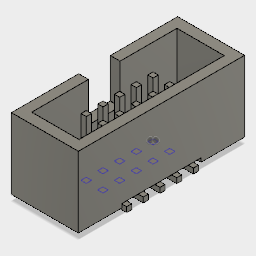
Gadgeteer Socket v1 (Autodesk Fusion 360 design; units mm, degrees)
Autodesk Fusion 360 part; units mm, degrees
sketch "Sketch1" plane through (0, 0, 0) normal (0, 1, 0) x (1, 0, 0)
  line L0 (2.55, 6.325) -> (-2.55, 6.325)
  line L1 (-2.55, 6.325) -> (-2.55, -6.325)
  line L2 (-2.55, -6.325) -> (2.55, -6.325)
  line L3 (2.55, -6.325) -> (2.55, 6.325)
  line L4 (2.55, 6.325) -> (-2.55, -6.325) construction
  line L5 (-2.55, 6.325) -> (2.55, -6.325) construction
  line L6 (1.8, 5.525) -> (-1.8, 5.525)
  line L7 (-1.8, 5.525) -> (-1.8, -5.525)
  line L8 (-1.8, -5.525) -> (1.8, -5.525)
  line L9 (1.8, -5.525) -> (1.8, 5.525)
  line L10 (1.8, 5.525) -> (-1.8, -5.525) construction
  line L11 (-1.8, 5.525) -> (1.8, -5.525) construction
  dimension "d1" = 12.65
  dimension "d2" = 5.1
  dimension "d3" = 3.6
  dimension "d4" = 11.05
  constraint perpendicular L0 L1
  constraint parallel L0 L2
  constraint parallel L1 L3
  constraint horizontal L0
  constraint coincident L4
  constraint coincident L5
  constraint perpendicular L6 L7
  constraint parallel L6 L8
  constraint parallel L7 L9
  constraint horizontal L6
  constraint coincident L10
  constraint coincident L11
extrude "Extrude1" add sketch "Sketch1" along normal blind 5.4 makes body 1
sketch "Sketch2" plane through (0, 5.4, 0) normal (0, 1, 0) x (-1, 0, 0)
  line L0 (-1.8, -5.525) -> (-1.8, 5.525)
  line L1 (-1.8, 5.525) -> (1.8, 5.525)
  line L2 (1.8, 5.525) -> (1.8, -5.525)
  line L3 (1.8, -5.525) -> (-1.8, -5.525)
  line L4 (-2.55, 6.325) -> (-2.55, -6.325)
  line L5 (-2.55, -6.325) -> (2.55, -6.325)
  line L6 (2.55, -6.325) -> (2.55, 6.325)
  line L7 (2.55, 6.325) -> (-2.55, 6.325)
  line L8 (1.8, 0) -> (2.55, 0)
  line L9 (1.8, -1.2) -> (2.55, -1.2)
  line L10 (2.55, -1.2) -> (2.55, 1.2)
  line L11 (2.55, 1.2) -> (1.8, 1.2)
  line L12 (1.8, 1.2) -> (1.8, -1.2)
  line L13 (1.8, -1.2) -> (2.55, 1.2) construction
  line L14 (2.55, -1.2) -> (1.8, 1.2) construction
  dimension "d7" = 2.4
  constraint midpoint L2
  constraint midpoint L6
  constraint perpendicular L9 L10
  constraint parallel L9 L11
  constraint parallel L10 L12
  constraint horizontal L9
  constraint coincident L13
  constraint coincident L14
  constraint midpoint L8
extrude "Extrude2" cut sketch "Sketch2" against normal blind 3 contours L2 L6 L8 L9 L10 L12 | L2 L6 L8 L10 L11 L12 bodies 1
extrude "Extrude3" add sketch "Sketch1" along normal blind 1 contours L6 L7 L8 L9 bodies 1
sketch "Sketch3" plane through (0, 0, 0) normal (0, 1, 0) x (1, 0, 0)
  line L0 (-0.835, 2.74) -> (-0.435, 2.74)
  line L1 (-0.435, 2.74) -> (-0.435, 2.34)
  line L2 (-0.435, 2.34) -> (-0.835, 2.34)
  line L3 (-0.835, 2.34) -> (-0.835, 2.74)
  line L4 (0.835, 2.74) -> (0.835, 2.34)
  line L5 (0.435, 2.74) -> (0.835, 2.74)
  line L6 (0.835, 2.34) -> (0.435, 2.34)
  line L7 (0.435, 2.34) -> (0.435, 2.74)
  line L8 (-0.435, 1.47) -> (-0.435, 1.07)
  line L9 (-0.835, 1.47) -> (-0.435, 1.47)
  line L10 (-0.435, 1.07) -> (-0.835, 1.07)
  line L11 (-0.835, 1.07) -> (-0.835, 1.47)
  line L12 (0.835, 1.47) -> (0.835, 1.07)
  line L13 (0.435, 1.47) -> (0.835, 1.47)
  line L14 (0.835, 1.07) -> (0.435, 1.07)
  line L15 (0.435, 1.07) -> (0.435, 1.47)
  line L16 (-0.435, 0.2) -> (-0.435, -0.2)
  line L17 (-0.835, 0.2) -> (-0.435, 0.2)
  line L18 (-0.435, -0.2) -> (-0.835, -0.2)
  line L19 (-0.835, -0.2) -> (-0.835, 0.2)
  line L20 (0.835, 0.2) -> (0.835, -0.2)
  line L21 (0.435, 0.2) -> (0.835, 0.2)
  line L22 (0.835, -0.2) -> (0.435, -0.2)
  line L23 (0.435, -0.2) -> (0.435, 0.2)
  line L24 (-0.435, -1.07) -> (-0.435, -1.47)
  line L25 (-0.835, -1.07) -> (-0.435, -1.07)
  line L26 (-0.435, -1.47) -> (-0.835, -1.47)
  line L27 (-0.835, -1.47) -> (-0.835, -1.07)
  line L28 (0.835, -1.07) -> (0.835, -1.47)
  line L29 (0.435, -1.07) -> (0.835, -1.07)
  line L30 (0.835, -1.47) -> (0.435, -1.47)
  line L31 (0.435, -1.47) -> (0.435, -1.07)
  line L32 (-0.435, -2.34) -> (-0.435, -2.74)
  line L33 (-0.835, -2.34) -> (-0.435, -2.34)
  line L34 (-0.435, -2.74) -> (-0.835, -2.74)
  line L35 (-0.835, -2.74) -> (-0.835, -2.34)
  line L36 (0.835, -2.34) -> (0.835, -2.74)
  line L37 (0.435, -2.34) -> (0.835, -2.34)
  line L38 (0.835, -2.74) -> (0.435, -2.74)
  line L39 (0.435, -2.74) -> (0.435, -2.34)
  dimension "d12" = 0.4
  dimension "d13" = 0.4
  dimension "d16" = 1.27
  dimension "d17" = -5.08
  dimension "d20" = 2.54
  dimension "d21" = 0.635
  constraint horizontal L0
  constraint vertical L1
  constraint horizontal L2
  constraint vertical L3
  constraint midpoint L3
  constraint midpoint L0
extrude "Extrude4" add sketch "Sketch3" along normal blind 4.4 separate body makes body 2 at (0.5683, 1.4667, -0.2) makes body 3 at (0.835, 1.4667, -1.3367) makes body 4 at (0.835, 1.4667, 1.2033) makes body 5 at (-0.435, 1.4667, 2.4733) makes body 6 at (-0.7017, 1.4667, -0.2) makes body 7 at (0.835, 1.4667, 2.4733) makes body 8 at (-0.435, 1.4667, 1.2033) makes body 9 at (-0.435, 1.4667, -1.3367) makes body 10 at (-0.7017, 1.4667, -2.74) makes body 11 at (0.5683, 1.4667, -2.74)
extrude "Extrude5" add sketch "Sketch3" against normal blind 0.4 separate body makes body 12 at (0.7017, -0.2667, -2.74) makes body 13 at (0.5683, 0, 1.2033) makes body 14 at (0.5683, 0, 2.4733) makes body 15 at (0.5683, 0, -1.3367) makes body 16 at (-0.7017, -0.1333, -2.74) makes body 17 at (-0.435, -0.2667, 2.6067) makes body 18 at (-0.435, -0.2667, 1.3367) makes body 19 at (-0.5683, -0.2667, -0.2) makes body 20 at (-0.435, -0.2667, -1.2033) makes body 21 at (0.7017, -0.2667, -0.2)
sketch "Sketch4" plane through (2.55, 0, 0) normal (1, 0, 0) x (0, 0, -1)
  line L0 (-6.325, 0) -> (6.325, 0)
  line L1 (6.325, 0) -> (6.325, 5.4)
  line L2 (6.325, 5.4) -> (-6.325, 5.4)
  line L3 (-6.325, 5.4) -> (-6.325, 0)
  line L4 (-3, 0) -> (3, 0)
  line L5 (3, 0) -> (3, 0.3)
  line L6 (3, 0.3) -> (-3, 0.3)
  line L7 (-3, 0.3) -> (-3, 0)
  dimension "d26" = 6
  dimension "d27" = 0.3
  constraint horizontal L4
  constraint vertical L5
  constraint horizontal L6
  constraint vertical L7
  constraint coincident L0
extrude "Extrude6" cut sketch "Sketch4" against normal blind 5.1 contours L0 L4 L5 L6 L7 bodies 1
move_face "OffsetFaces1" offset 1.8 5 faces at (-0.835, -0.2667, 2.4733) (-0.835, -0.2667, 1.2033) (-0.835, -0.2667, -1.3367) (-0.835, -0.1333, 0.0667) (-0.835, -0.1333, -2.4733) on bodies 16 17 18 19 20
move_face "OffsetFaces2" offset 1.8 5 faces at (0.835, -0.1333, -0.0667) (0.835, -0.2667, 2.6067) (0.835, -0.2667, -1.2033) (0.835, -0.1333, -2.6067) (0.835, -0.2667, 1.3367) on bodies 12 13 14 15 21
